Autodesk Inventor part; units mm, degrees
(part 2 of 2)
  line L380 (-0.5258, 0.0291) -> (-0.4758, 0.0123)
  line L381 (-0.4758, 0.0123) -> (-0.4708, 0.0169)
  line L382 (-0.4708, 0.0169) -> (-0.4661, 0.0215)
  line L383 (-0.4661, 0.0215) -> (-0.4617, 0.0263)
  line L384 (-0.4617, 0.0263) -> (-0.4575, 0.0311)
  line L385 (-0.4575, 0.0311) -> (-0.4535, 0.036)
  line L386 (-0.4535, 0.036) -> (-0.4498, 0.041)
  line L387 (-0.4498, 0.041) -> (-0.4464, 0.0461)
  line L388 (-0.4464, 0.0461) -> (-0.4433, 0.0513)
  line L389 (-0.4433, 0.0513) -> (-0.4405, 0.0565)
  line L390 (-0.4405, 0.0565) -> (-0.4381, 0.0618)
  line L391 (-0.4381, 0.0618) -> (-0.4363, 0.0672)
  line L392 (-0.4363, 0.0672) -> (-0.435, 0.0727)
  line L393 (-0.435, 0.0727) -> (-0.4341, 0.0754)
  line L394 (-0.4341, 0.0754) -> (-0.4329, 0.0781)
  line L395 (-0.4329, 0.0781) -> (-0.4316, 0.0807)
  line L396 (-0.4316, 0.0807) -> (-0.4308, 0.082)
  line L397 (-0.4308, 0.082) -> (-0.4298, 0.0833)
  line L398 (-0.4298, 0.0833) -> (-0.4287, 0.0845)
  line L399 (-0.4287, 0.0845) -> (-0.4274, 0.0858)
  line L400 (-0.4274, 0.0858) -> (-0.4257, 0.0869)
  line L401 (-0.4257, 0.0869) -> (-0.4215, 0.0877)
  line L402 (-0.4215, 0.0877) -> (-0.3984, 0.0853)
  line L403 (-0.3984, 0.0853) -> (-0.3752, 0.0848)
  line L404 (-0.3752, 0.0848) -> (-0.3712, 0.0835)
  line L405 (-0.3712, 0.0835) -> (-0.3696, 0.0821)
  line L406 (-0.3696, 0.0821) -> (-0.3684, 0.0807)
  line L407 (-0.3684, 0.0807) -> (-0.3675, 0.0794)
  line L408 (-0.3675, 0.0794) -> (-0.3667, 0.078)
  line L409 (-0.3667, 0.078) -> (-0.3661, 0.0766)
  line L410 (-0.3661, 0.0766) -> (-0.3651, 0.0738)
  line L411 (-0.3651, 0.0738) -> (-0.3643, 0.071)
  line L412 (-0.3643, 0.071) -> (-0.3638, 0.0682)
  line L413 (-0.3638, 0.0682) -> (-0.3631, 0.0626)
  line L414 (-0.3631, 0.0626) -> (-0.362, 0.057)
  line L415 (-0.362, 0.057) -> (-0.3603, 0.0514)
  line L416 (-0.3603, 0.0514) -> (-0.3582, 0.0459)
  line L417 (-0.3582, 0.0459) -> (-0.3557, 0.0404)
  line L418 (-0.3557, 0.0404) -> (-0.353, 0.0349)
  line L419 (-0.353, 0.0349) -> (-0.3499, 0.0295)
  line L420 (-0.3499, 0.0295) -> (-0.3466, 0.0241)
  line L421 (-0.3466, 0.0241) -> (-0.3431, 0.0188)
  line L422 (-0.3431, 0.0188) -> (-0.3392, 0.0135)
  line L423 (-0.3392, 0.0135) -> (-0.3351, 0.0083)
  line L424 (-0.3351, 0.0083) -> (-0.3308, 0.0032)
  line L425 (-0.3308, 0.0032) -> (-0.2791, 0.0136)
  line L426 (-0.2791, 0.0136) -> (-0.2771, 0.02)
  line L427 (-0.2771, 0.02) -> (-0.2754, 0.0264)
  line L428 (-0.2754, 0.0264) -> (-0.2739, 0.0328)
  line L429 (-0.2739, 0.0328) -> (-0.2727, 0.0391)
  line L430 (-0.2727, 0.0391) -> (-0.2717, 0.0453)
  line L431 (-0.2717, 0.0453) -> (-0.271, 0.0515)
  line L432 (-0.271, 0.0515) -> (-0.2706, 0.0576)
  line L433 (-0.2706, 0.0576) -> (-0.2705, 0.0636)
  line L434 (-0.2705, 0.0636) -> (-0.2707, 0.0695)
  line L435 (-0.2707, 0.0695) -> (-0.2713, 0.0753)
  line L436 (-0.2713, 0.0753) -> (-0.2724, 0.0809)
  line L437 (-0.2724, 0.0809) -> (-0.274, 0.0863)
  line L438 (-0.274, 0.0863) -> (-0.2746, 0.0891)
  line L439 (-0.2746, 0.0891) -> (-0.2749, 0.092)
  line L440 (-0.2749, 0.092) -> (-0.2751, 0.0949)
  line L441 (-0.2751, 0.0949) -> (-0.275, 0.0965)
  line L442 (-0.275, 0.0965) -> (-0.2748, 0.098)
  line L443 (-0.2748, 0.098) -> (-0.2745, 0.0997)
  line L444 (-0.2745, 0.0997) -> (-0.274, 0.1014)
  line L445 (-0.274, 0.1014) -> (-0.2731, 0.1033)
  line L446 (-0.2731, 0.1033) -> (-0.2699, 0.106)
  line L447 (-0.2699, 0.106) -> (-0.2487, 0.1155)
  line L448 (-0.2487, 0.1155) -> (-0.2283, 0.1267)
  line L449 (-0.2283, 0.1267) -> (-0.2241, 0.1276)
  line L450 (-0.2241, 0.1276) -> (-0.2221, 0.1272)
  line L451 (-0.2221, 0.1272) -> (-0.2204, 0.1266)
  line L452 (-0.2204, 0.1266) -> (-0.2189, 0.1258)
  line L453 (-0.2189, 0.1258) -> (-0.2176, 0.125)
  line L454 (-0.2176, 0.125) -> (-0.2163, 0.1241)
  line L455 (-0.2163, 0.1241) -> (-0.214, 0.1222)
  line L456 (-0.214, 0.1222) -> (-0.212, 0.1202)
  line L457 (-0.212, 0.1202) -> (-0.2101, 0.1181)
  line L458 (-0.2101, 0.1181) -> (-0.2067, 0.1135)
  line L459 (-0.2067, 0.1135) -> (-0.2029, 0.1092)
  line L460 (-0.2029, 0.1092) -> (-0.1987, 0.1053)
  line L461 (-0.1987, 0.1053) -> (-0.1941, 0.1015)
  line L462 (-0.1941, 0.1015) -> (-0.1892, 0.098)
  line L463 (-0.1892, 0.098) -> (-0.1841, 0.0946)
  line L464 (-0.1841, 0.0946) -> (-0.1788, 0.0914)
  line L465 (-0.1788, 0.0914) -> (-0.1732, 0.0884)
  line L466 (-0.1732, 0.0884) -> (-0.1675, 0.0856)
  line L467 (-0.1675, 0.0856) -> (-0.1615, 0.083)
  line L468 (-0.1615, 0.083) -> (-0.1554, 0.0805)
  line L469 (-0.1554, 0.0805) -> (-0.1491, 0.0782)
  line L470 (-0.1491, 0.0782) -> (-0.1095, 0.1131)
  line L471 (-0.1095, 0.1131) -> (-0.111, 0.1196)
  line L472 (-0.111, 0.1196) -> (-0.1127, 0.126)
  line L473 (-0.1127, 0.126) -> (-0.1146, 0.1323)
  line L474 (-0.1146, 0.1323) -> (-0.1166, 0.1383)
  line L475 (-0.1166, 0.1383) -> (-0.1189, 0.1442)
  line L476 (-0.1189, 0.1442) -> (-0.1214, 0.1499)
  line L477 (-0.1214, 0.1499) -> (-0.1241, 0.1554)
  line L478 (-0.1241, 0.1554) -> (-0.127, 0.1607)
  line L479 (-0.127, 0.1607) -> (-0.1301, 0.1657)
  line L480 (-0.1301, 0.1657) -> (-0.1335, 0.1704)
  line L481 (-0.1335, 0.1704) -> (-0.1373, 0.1747)
  line L482 (-0.1373, 0.1747) -> (-0.1414, 0.1786)
  line L483 (-0.1414, 0.1786) -> (-0.1433, 0.1807)
  line L484 (-0.1433, 0.1807) -> (-0.1451, 0.183)
  line L485 (-0.1451, 0.183) -> (-0.1466, 0.1855)
  line L486 (-0.1466, 0.1855) -> (-0.1474, 0.1869)
  line L487 (-0.1474, 0.1869) -> (-0.148, 0.1883)
  line L488 (-0.148, 0.1883) -> (-0.1485, 0.1899)
  line L489 (-0.1485, 0.1899) -> (-0.1489, 0.1917)
  line L490 (-0.1489, 0.1917) -> (-0.1491, 0.1937)
  line L491 (-0.1491, 0.1937) -> (-0.1477, 0.1978)
  line L492 (-0.1477, 0.1978) -> (-0.1341, 0.2166)
  line L493 (-0.1341, 0.2166) -> (-0.122, 0.2364)
  line L494 (-0.122, 0.2364) -> (-0.1188, 0.2392)
  line L495 (-0.1188, 0.2392) -> (-0.1169, 0.2399)
  line L496 (-0.1169, 0.2399) -> (-0.1151, 0.2402)
  line L497 (-0.1151, 0.2402) -> (-0.1134, 0.2403)
  line L498 (-0.1134, 0.2403) -> (-0.1119, 0.2403)
  line L499 (-0.1119, 0.2403) -> (-0.1103, 0.2402)
  line L500 (-0.1103, 0.2402) -> (-0.1074, 0.2397)
  line L501 (-0.1074, 0.2397) -> (-0.1046, 0.239)
  line L502 (-0.1046, 0.239) -> (-0.1019, 0.238)
  line L503 (-0.1019, 0.238) -> (-0.0967, 0.2358)
  line L504 (-0.0967, 0.2358) -> (-0.0913, 0.234)
  line L505 (-0.0913, 0.234) -> (-0.0856, 0.2327)
  line L506 (-0.0856, 0.2327) -> (-0.0798, 0.2317)
  line L507 (-0.0798, 0.2317) -> (-0.0738, 0.2311)
  line L508 (-0.0738, 0.2311) -> (-0.0677, 0.2307)
  line L509 (-0.0677, 0.2307) -> (-0.0615, 0.2306)
  line L510 (-0.0615, 0.2306) -> (-0.0552, 0.2308)
  line L511 (-0.0552, 0.2308) -> (-0.0488, 0.2313)
  line L512 (-0.0488, 0.2313) -> (-0.0423, 0.2319)
  line L513 (-0.0423, 0.2319) -> (-0.0357, 0.2329)
  line L514 (-0.0357, 0.2329) -> (-0.0291, 0.234)
  line L515 (-0.0291, 0.234) -> (-0.0123, 0.284)
  line L516 (-0.0123, 0.284) -> (-0.0169, 0.2889)
  line L517 (-0.0169, 0.2889) -> (-0.0215, 0.2936)
  line L518 (-0.0215, 0.2936) -> (-0.0263, 0.2981)
  line L519 (-0.0263, 0.2981) -> (-0.0311, 0.3023)
  line L520 (-0.0311, 0.3023) -> (-0.036, 0.3063)
  line L521 (-0.036, 0.3063) -> (-0.041, 0.31)
  line L522 (-0.041, 0.31) -> (-0.0461, 0.3134)
  line L523 (-0.0461, 0.3134) -> (-0.0513, 0.3165)
  line L524 (-0.0513, 0.3165) -> (-0.0565, 0.3193)
  line L525 (-0.0565, 0.3193) -> (-0.0618, 0.3216)
  line L526 (-0.0618, 0.3216) -> (-0.0672, 0.3234)
  line L527 (-0.0672, 0.3234) -> (-0.0727, 0.3248)
  line L528 (-0.0727, 0.3248) -> (-0.0754, 0.3257)
  line L529 (-0.0754, 0.3257) -> (-0.0781, 0.3268)
  line L530 (-0.0781, 0.3268) -> (-0.0807, 0.3282)
  line L531 (-0.0807, 0.3282) -> (-0.082, 0.329)
  line L532 (-0.082, 0.329) -> (-0.0833, 0.3299)
  line L533 (-0.0833, 0.3299) -> (-0.0845, 0.331)
  line L534 (-0.0845, 0.331) -> (-0.0858, 0.3323)
  line L535 (-0.0858, 0.3323) -> (-0.0869, 0.3341)
  line L536 (-0.0869, 0.3341) -> (-0.0877, 0.3382)
  line L537 (-0.0877, 0.3382) -> (-0.0853, 0.3614)
  line L538 (-0.0853, 0.3614) -> (-0.0848, 0.3846)
  line L539 (-0.0848, 0.3846) -> (-0.0835, 0.3886)
  point P0 (0, 0)
body "Solid1"
